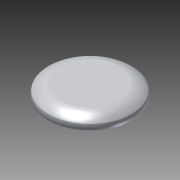
# Autodesk Inventor part: 3061Frisbee
Saved by Autodesk Inventor 2013 (Build 170138000, 138)
## iProperties
Created: 2013-01-12
Part Number: 3061Frisbee
Material: Generic
Document SubType Name: Modeling
Designer: dadegenhardt
Density: 1 g/cm^3
Author: dadegenhardt
Autodesk Inventor part; units mm, degrees
ref_plane "YZ Plane" through (0, 0, 0) normal (1, 0, 0) x (0, 1, 0)
ref_plane "XZ Plane" through (0, 0, 0) normal (0, 1, 0) x (-1, 0, 0)
ref_plane "XY Plane" through (0, 0, 0) normal (0, 0, 1) x (1, 0, 0)
sketch "Sketch1" plane through (0, 0, 0) normal (0, 1, 0) x (-1, 0, 0)
  circle A0 centre (0, 0) radius 97.6313
  dimension "d1" = 195.2625
  constraints: 1 centre point, 1 coincident
  measures "d1" diameter of A0
extrude "Extrusion1" add sketch "Sketch1" along normal blind 2.3813
sketch "Sketch2" plane through (0, 0, 0) normal (0, 0, 1) x (1, 0, 0)
  line L0 (97.6313, 2.3813) -> (-97.6313, 2.3813) projected
  line L1 (-97.6313, 0) -> (97.6313, 0) projected
  line L2 (97.6313, 2.3813) -> (97.6313, 0)
  line L3 (97.6313, 2.3813) -> (97.6313, -16.6688)
  arc A0 (137.2553, -16.6688) -> (97.6313, 2.3813) centre (86.0498, -72.4422) ccw
  arc A1 (132.1753, -16.6687) -> (97.6313, 0) centre (89.5948, -60.7831) ccw
  line L4 (0, 2.3813) -> (0, -35.7188)
  line L5 (137.2552, -35.7188) -> (132.1752, -35.7188)
  arc A2 (132.1752, -35.7188) -> (132.1753, -16.6687) centre (104.394, -26.1937) ccw
  arc A3 (137.2552, -35.7188) -> (137.2553, -16.6688) centre (109.474, -26.1937) ccw
  point P0 (0, 0)
  dimension "d14" = 19.05
  constraints: 8 end point, 8 point on circle, 4 centre point, 1 midpoint, 1 perpendicular
  measures "d14" distance of L0.start L3.end
revolve "Revolution1" add sketch "Sketch2" angle 360 about axis through (0, 2.3813, 0) along (0, -1, 0) contours A0 A3 L5 A2 A1 L2
fillet "Fillet1" radius 3.175 1 edges at (-137.2553, -16.6687, 0)
fillet "Fillet2" radius 1.27 1 edges at (-137.2553, -35.7187, 0)
fillet "Fillet3" radius 1.27 1 edges at (-97.6313, 2.3813, 0)
fillet "Fillet4" radius 1.27 1 edges at (-132.1753, -35.7187, 0)
body "Solid1"
